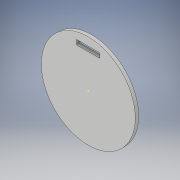
# Autodesk Inventor part: Light Ring Mount
Saved by Autodesk Inventor 2019 (Build 230136000, 136)
## iProperties
Created: 2019-01-11
Part Number: Light Ring Mount
Material: Generic
Document SubType Name: Modeling
Designer: pepin
Density: 1 g/cm^3
Appearance: Default
Author: pepin
Autodesk Inventor part; units mm, degrees
ref_plane "YZ Plane" through (0, 0, 0) normal (1, 0, 0) x (0, 1, 0)
ref_plane "XZ Plane" through (0, 0, 0) normal (0, 1, 0) x (-1, 0, 0)
ref_plane "XY Plane" through (0, 0, 0) normal (0, 0, 1) x (1, 0, 0)
sketch "Sketch1" plane through (0, 0, 0) normal (0, 0, 1) x (1, 0, 0)
  circle A0 centre (0, 0) radius 35
  dimension "d0" = 70
  constraints: 1 centre point, 1 coincident
  measures "d0" diameter of A0
extrude "Extrusion1" add sketch "Sketch1" along normal blind 2.54
sketch "Sketch2" plane through (0, 0, 2.54) normal (0, 0, 1) x (1, 0, 0)
  line L0 (0, 0) -> (0, 34.7042) construction
  line L1 (-8.676, 28.9646) -> (8.676, 28.9646)
  line L2 (8.676, 28.9646) -> (8.676, 25.4646)
  line L3 (8.676, 25.4646) -> (-8.676, 25.4646)
  line L4 (-8.676, 25.4646) -> (-8.676, 28.9646)
  line L5 (-8.676, 28.9646) -> (8.676, 25.4646) construction
  line L6 (8.676, 28.9646) -> (-8.676, 25.4646) construction
  point P0 (0, 27.2146)
  dimension "d3" = 17.3521
  dimension "d4" = 3.5
  constraints: 14 end point, 2 midpoint, 2 parallel, 2 perpendicular, 1 point on line, 1 vertical
  measures "d3" distance of L1.start L1.end
  measures "d4" distance of L1.end L2.end
extrude "Extrusion2" cut sketch "Sketch2" against normal blind 2.54
sketch "Sketch3" plane through (0, 0, 2.54) normal (0, 0, 1) x (1, 0, 0)
  point P0 (0, 0)
body "Solid1"
